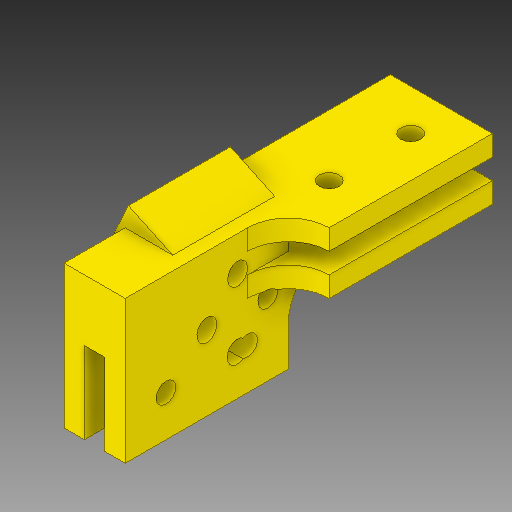
# Autodesk Inventor part: trsthrustmt2
Saved by Autodesk Inventor 2018.1 (Build 221171000, 171)
## iProperties
Created: 2017-08-13
Part Number: trsthrustmt2
Material: Generic
Document SubType Name: Modeling
Designer: Kai
Density: 1 g/cm^3
Appearance: Default
Author: Kai
Autodesk Inventor part; units mm, degrees
ref_plane "YZ Plane" through (0, 0, 0) normal (1, 0, 0) x (0, 1, 0)
ref_plane "XZ Plane" through (0, 0, 0) normal (0, 1, 0) x (-1, 0, 0)
ref_plane "XY Plane" through (0, 0, 0) normal (0, 0, 1) x (1, 0, 0)
sketch "Sketch1" plane through (0, 0, 0) normal (0, 0, 1) x (1, 0, 0)
  line L0 (12.7, 9.525) -> (-19.05, 9.525)
  line L1 (-19.05, 9.525) -> (-19.05, -9.525)
  line L2 (-19.05, -9.525) -> (12.7, -9.525)
  line L3 (12.7, -9.525) -> (12.7, -3.175)
  line L4 (12.7, -3.175) -> (-12.7, -3.175)
  line L5 (-12.7, -3.175) -> (-12.7, 3.175)
  line L6 (-12.7, 3.175) -> (12.7, 3.175)
  line L7 (12.7, 3.175) -> (12.7, 9.525)
  line L8 (0, 0) -> (-2.6418, 0) construction
  dimension "d0" = 31.75
  dimension "d1" = 19.05
  dimension "d2" = 6.35
  dimension "d3" = 25.4
  dimension "d4" = 6.35
  constraints: 18 end point, 7 perpendicular, 2 horizontal, 1 point on line, 1 other
  measures "d0" distance of L0.start L0.end
  measures "d1" distance of L0.end L1.end
  measures "d2" distance of L2.end L3.end
  measures "d3" distance of L3.end L4.end
  measures "d4" distance of L4.end L5.end
extrude "Extrusion1" add sketch "Sketch1" along normal blind 50.8
sketch "Sketch2" plane through (0, 0, 50.8) normal (0, 0, 1) x (1, 0, 0)
  line L0 (-19.05, 9.525) -> (-19.05, -9.525) projected
  line L1 (-19.05, -9.525) -> (-12.7, -9.525)
  line L2 (-12.7, 34.925) -> (-19.05, 34.925)
  line L3 (-19.05, 34.925) -> (-19.05, -9.525)
  line L4 (0, 3.175) -> (0, 34.925)
  line L5 (0, 34.925) -> (-6.35, 34.925)
  line L6 (-6.35, 34.925) -> (-6.35, 9.525)
  line L7 (-6.35, 9.525) -> (-12.7, 9.525)
  line L8 (-12.7, 9.525) -> (-12.7, 34.925)
  line L9 (-12.7, -9.525) -> (0, -9.525)
  line L10 (0, 3.175) -> (0, -9.525)
  point P0 (0, 0)
  dimension "d7" = 6.35
  dimension "d8" = 44.45
  dimension "d9" = 6.35
  constraints: 20 end point, 3 parallel, 1 horizontal, 1 perpendicular, 1 point on line
  measures "d7" distance of L2.end L2.start
  measures "d8" distance of L2.start L1.end
  measures "d9" distance of L5.end L4.end
extrude "Extrusion2" add sketch "Sketch2" along normal blind 50.8
fillet "Fillet1" radius 12.7 2 edges at (0, -6.35, 50.8) (0, 6.35, 50.8)
fillet "Fillet2" radius 12.7 2 edges at (-3.175, 9.525, 50.8) (-15.875, 9.525, 50.8)
sketch "Sketch3" plane through (0, 0, 50.8) normal (0, 0, -1) x (-1, 0, 0)
  line L0 (19.05, 22.225) -> (12.7, 22.225) projected
  line L1 (19.05, 22.225) -> (4.2447, -9.525)
  line L2 (19.05, -9.525) -> (0, -9.525) projected
  line L3 (19.05, 22.225) -> (54.0822, 22.225) construction
  line L4 (4.2447, -9.525) -> (18.0569, -15.9657)
  line L5 (18.0569, -15.9657) -> (32.8621, 15.7843)
  line L6 (32.8621, 15.7843) -> (19.05, 22.225)
  point P0 (0, 0)
  dimension "d15" = 115
  dimension "d16" = 15.24
  constraints: 10 end point, 3 perpendicular, 1 equal length, 1 horizontal, 1 point on line
  measures "d15" angle of L1 L3
  measures "d16" distance of L1.end L4.end
extrude "Extrusion3" add sketch "Sketch3" against normal blind 31.75
sketch "Sketch4" plane through (0, -3.175, 50.8) normal (1, 0, 0) x (0, 0, -1)
  circle A0 centre (-12.7, 25.4) radius 3.1
  line L0 (0, 38.1) -> (-50.8, 38.1) projected
  line L1 (0, 25.4) -> (0, 38.1) projected
  circle A1 centre (-38.1, 25.4) radius 3.1
  point P0 (50.8, 3.175)
  dimension "d19" = 6.2
  dimension "d20" = 12.7
  dimension "d21" = 12.7
  dimension "d22" = 6.2
  dimension "d23" = 25.4
  constraints: 2 centre point
  measures "d19" diameter of A0
  measures "d20" distance from line of L0 A0.centre
  measures "d21" distance from line of L1 A0.centre
  measures "d22" diameter of A1
  measures "d23" distance of A0.centre A1.centre
extrude "Extrusion4" cut sketch "Sketch4" against normal blind 31.75
sketch "Sketch5" plane through (-19.05, -9.525, 0) normal (0, -1, 0) x (1, 0, 0)
  circle A0 centre (19.05, 12.7) radius 3.1
  line L0 (31.75, 0) -> (31.75, 50.8) projected
  line L1 (0, 0) -> (31.75, 0) projected
  circle A1 centre (19.05, 38.1) radius 3.1
  point P0 (19.05, 0)
  dimension "d26" = 6.2
  dimension "d27" = 12.7
  dimension "d28" = 12.7
  dimension "d29" = 6.2
  dimension "d30" = 25.4
  constraints: 2 centre point
  measures "d26" diameter of A0
  measures "d27" distance from line of L0 A0.centre
  measures "d28" distance from line of L1 A0.centre
  measures "d29" diameter of A1
  measures "d30" distance of A1.centre A0.centre
extrude "Extrusion5" cut sketch "Sketch5" against normal blind 31.75
sketch "Sketch6" plane through (-19.05, 9.525, 0) normal (0, 1, 0) x (1, 0, 0)
  arc A0 (19.05, -41.2) -> (15.95, -38.1) centre (19.05, -38.1) ccw projected
  circle A1 centre (19.05, -38.1) radius 6
  point P0 (19.05, 0)
  dimension "d33" = 12
  constraints: 1 centre point, 1 coincident
  measures "d33" diameter of A1
sketch "Sketch7" plane through (-19.05, -9.525, 101.6) normal (-1, 0, 0) x (0, 0, 1)
  circle A0 centre (-38.1, 31.75) radius 3.1 projected
  circle A1 centre (-38.1, 31.75) radius 6
  point P0 (-101.6, 9.525)
  dimension "d34" = 12
  constraints: 1 centre point, 1 coincident
  measures "d34" diameter of A1
extrude "Extrusion6" cut sketch "Sketch7" along normal blind 31.75
extrude "Extrusion7" cut sketch "Sketch6" along normal blind 31.75
sketch "Sketch8" plane through (-18.0569, -15.9657, 50.8) normal (-0.9063078, -0.4226183, 0) x (0, 0, 1)
  line L0 (0, 35.0322) -> (31.75, 35.0322) projected
  line L1 (0, 0) -> (31.75, 0) projected
  line L2 (31.75, 35.0322) -> (0, 0) construction
  circle A0 centre (15.875, 17.5161) radius 9.5 construction
  circle A1 centre (15.8, 8.0164) radius 1.6
  circle A2 centre (25.3747, 17.4411) radius 1.6
  circle A3 centre (15.95, 27.0158) radius 1.6
  circle A4 centre (6.3753, 17.5911) radius 1.6
  point P0 (-50.8, 6.8387)
  dimension "d40" = 19
  dimension "d41" = 3.2
  dimension "d44" = 360
  constraints: 4 centre point, 2 end point, 1 midpoint, 12 other
  measures "d41" diameter of A1
extrude "Extrusion8" cut sketch "Sketch8" against normal blind 76.2
ref_plane "Work Plane1" through (-12.3018, -13.2821, 50.8) normal (-0.9063078, -0.4226183, 0) x (0, 0, 1)
sketch "Sketch9" plane through (-12.3018, -13.2821, 50.8) normal (-0.9063078, -0.4226183, 0) x (0, 0, 1)
  arc A0 (15.3548, 25.5307) -> (15.3181, 28.4858) centre (15.95, 27.0158) ccw projected
  circle A1 centre (15.95, 27.0158) radius 3.1
  circle A2 centre (25.3747, 17.4411) radius 1.6 projected
  circle A3 centre (25.3747, 17.4411) radius 3.1
  circle A4 centre (15.8, 8.0164) radius 1.6 projected
  circle A5 centre (15.8, 8.0164) radius 3.1
  circle A6 centre (6.3753, 17.5911) radius 1.6 projected
  circle A7 centre (6.3753, 17.5911) radius 3.1
  point P0 (-50.8, 6.8387)
  dimension "d49" = 6.2
  dimension "d50" = 6.2
  dimension "d51" = 6.2
  dimension "d52" = 6.2
  constraints: 4 centre point, 4 coincident
  measures "d49" diameter of A1
  measures "d50" diameter of A3
  measures "d51" diameter of A5
  measures "d52" diameter of A7
extrude "Extrusion9" cut sketch "Sketch9" against normal blind 76.2
mirror "Mirror1" about plane through (-12.7, 34.925, 50.8) normal (0, 1, 0) remove original yes
body "Solid1"
